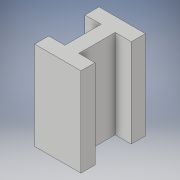
# Autodesk Inventor part: testh
Saved by Autodesk Inventor 2018 (Build 220112000, 112)
## iProperties
Created: 2018-04-30
Part Number: testh
Material: Generic
Document SubType Name: Modeling
Designer: 4070609
Density: 1 g/cm^3
Appearance: Default
Author: 4070609
Autodesk Inventor part; units mm, degrees
ref_plane "YZ Plane" through (0, 0, 0) normal (1, 0, 0) x (0, 1, 0)
ref_plane "XZ Plane" through (0, 0, 0) normal (0, 1, 0) x (-1, 0, 0)
ref_plane "XY Plane" through (0, 0, 0) normal (0, 0, 1) x (1, 0, 0)
sketch "Sketch1" plane through (0, 0, 0) normal (0, 1, 0) x (-1, 0, 0)
  line L0 (0, 0) -> (9.2, 0)
  line L1 (9.2, 0) -> (9.2, -12.8)
  line L2 (9.2, -12.8) -> (0, -12.8)
  line L3 (0, -12.8) -> (0, 0)
  line L4 (9.2, -12.8) -> (9.2, -10)
  line L5 (9.2, -10) -> (6, -10)
  line L6 (6, -10) -> (6, -2.8)
  line L7 (6, -2.8) -> (9.2, -2.8)
  line L8 (9.2, -2.8) -> (9.2, -10)
  line L9 (0, 0) -> (0, -2.8)
  line L10 (0, -2.8) -> (3.2, -2.8)
  line L11 (3.2, -2.8) -> (3.2, -10)
  line L12 (3.2, -10) -> (0, -10)
  line L13 (0, -10) -> (0, -2.8)
  dimension "d0" = 9.2
  dimension "d1" = 12.8
  dimension "d2" = 2.8
  dimension "d3" = 3.2
  dimension "d4" = 7.2
  dimension "d5" = 3.2
  constraints: 28 end point, 6 parallel, 3 horizontal, 3 perpendicular, 2 point on line
  measures "d0" distance of L1.end L2.end
  measures "d1" distance of L0.end L1.end
  measures "d2" distance of L1.end L4.end
  measures "d3" distance of L6.end L7.end
  measures "d4" distance of L5.end L6.end
  measures "d5" distance of L11.end L12.end
extrude "Extrusion1" add sketch "Sketch1" along normal blind 17.6 contours L0 L1 L7 L6 L5 L2 L3 L12 L11 L10
body "Solid1"
